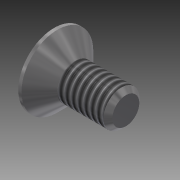
# Autodesk Inventor part: FHS4x8
Saved by Autodesk Inventor 2015 SP1 (Build 190203100, 203)
## iProperties
Category: Hardware
Created: 2015-01-27
Part Number: FHS4x8
Material: Steel, Alloy
Document SubType Name: Modeling
Designer: Jack
Density: 7.73 g/cm^3
Appearance: Semi-Polished
Vendor: McMaster Carr
Mass: 1.06716 g
Surface Area: 2.05053 cm^2
Volume: 0.138054 cm^3
Author: Jack
Title: FHS 4x8
Autodesk Inventor part; units mm, degrees
ref_plane "YZ Plane" through (0, 0, 0) normal (1, 0, 0) x (0, 1, 0)
ref_plane "XZ Plane" through (0, 0, 0) normal (0, 1, 0) x (-1, 0, 0)
ref_plane "XY Plane" through (0, 0, 0) normal (0, 0, 1) x (1, 0, 0)
sketch "Sketch1" plane through (0, 0, 0) normal (0, 0, 1) x (1, 0, 0)
  line L0 (0, 0) -> (0, 4)
  line L1 (0, 4) -> (0.36, 4)
  line L2 (0.36, 4) -> (2.36, 2)
  line L3 (2.36, 2) -> (8, 2)
  line L4 (8, 2) -> (8, 0)
  line L5 (8, 0) -> (0, 0)
  dimension "d0" = 4
  dimension "d1" = 0.36
  dimension "d2" = 135
  dimension "d3" = 8
  dimension "d4" = 2
  constraints: 12 end point, 3 horizontal, 2 vertical
  measures "d0" distance of L0.start L0.end
  measures "d1" distance of L0.end L1.end
  measures "d2" angle of L1 L2
  measures "d3" distance from line of L0 L3.end
  measures "d4" distance from line of L0.start L3
revolve "Revolution1" add sketch "Sketch1" angle 360 about axis through (8, 0, 0) along (-1, 0, 0)
chamfer "Chamfer1" distance 0.5 angle 45 1 edges at (8, -2, 0)
sketch "Sketch2" plane through (0, 0, 0) normal (-1, 0, 0) x (0, 0, 1)
  circle A0 centre (0, 0) radius 4 projected
  line L0 (-1.4434, 0) -> (-0.7217, 1.25)
  line L1 (-0.7217, 1.25) -> (0.7217, 1.25)
  line L2 (0.7217, 1.25) -> (1.4434, 0)
  line L3 (1.4434, 0) -> (0.7217, -1.25)
  line L4 (0.7217, -1.25) -> (-0.7217, -1.25)
  line L5 (-0.7217, -1.25) -> (-1.4434, 0)
  dimension "d9" = 2.5
  constraints: 12 end point, 1 coincident, 1 horizontal, 13 other
  measures "d9" distance between parallel lines of L1 L4
extrude "Extrusion1" cut sketch "Sketch2" against normal blind 1.5 contours L0 L1 L2 L3 L4 L5
thread "Thread1" size "M4x0.7" class "6g" standard "ANSI Metric M Profile" full length
body "Solid1"
